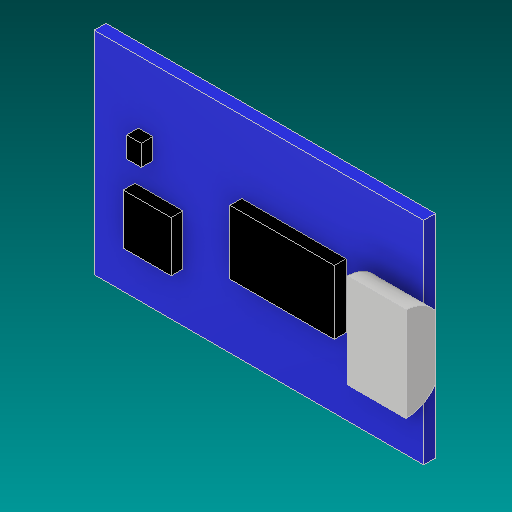
# Autodesk Inventor part: Regulador
Saved by Autodesk Inventor 2019 (Build 230136000, 136)
## iProperties
Created: 2020-01-17
Part Number: Regulador
Material: Generic
Document SubType Name: Modeling
Designer: Santiago
Density: 1 g/cm^3
Appearance: Default
Author: Santiago
Autodesk Inventor part; units mm, degrees
ref_plane "YZ Plane" through (0, 0, 0) normal (1, 0, 0) x (0, 1, 0)
ref_plane "XZ Plane" through (0, 0, 0) normal (0, 1, 0) x (-1, 0, 0)
ref_plane "XY Plane" through (0, 0, 0) normal (0, 0, 1) x (1, 0, 0)
sketch "Sketch1" plane through (0, 0, 0) normal (0, 0, 1) x (1, 0, 0)
  line L0 (0, 0) -> (28, 0)
  line L1 (28, 0) -> (28, 18)
  line L2 (28, 18) -> (0, 18)
  line L3 (0, 18) -> (0, 0)
  dimension "d0" = 28
  dimension "d1" = 18
  dimension "d2" = 28
  constraints: 8 end point, 2 perpendicular, 1 horizontal
  measures "d0" distance of L0.start L0.end
  measures "d1" distance of L0.end L1.end
  measures "d2" distance of L1.end L2.end
extrude "Extrusion1" add sketch "Sketch1" along normal blind 1
sketch "Sketch2" plane through (0, 0, 1) normal (0, 0, 1) x (1, 0, 0)
  line L0 (21.3992, 11.8771) -> (21.3992, 6.4359)
  line L1 (21.3992, 6.4359) -> (12.5353, 6.4359)
  line L2 (12.5353, 6.4359) -> (12.5353, 11.8771)
  line L3 (12.5353, 11.8771) -> (21.3992, 11.8771)
  line L4 (3.7591, 12.6669) -> (3.7591, 10.8901)
  line L5 (3.7591, 10.8901) -> (4.997, 10.8901)
  line L6 (4.997, 10.8901) -> (4.997, 12.6669)
  line L7 (4.997, 12.6669) -> (3.7591, 12.6669)
  line L8 (3.4697, 8.4681) -> (7.5353, 8.4681)
  line L9 (7.5353, 8.4681) -> (7.5353, 4.1843)
  line L10 (7.5353, 4.1843) -> (3.4697, 4.1843)
  line L11 (3.4697, 4.1843) -> (3.4697, 8.4681)
  point P0 (0, 0)
  constraints: 24 end point, 9 perpendicular, 2 vertical, 1 horizontal
extrude "Extrusion2" add sketch "Sketch2" along normal blind 1
sketch "Sketch3" plane through (28, 0, 0) normal (1, 0, 0) x (0, 0, -1)
  line L0 (-1, 6.4359) -> (-1, 11.8771) projected
  line L1 (-1, 9.1565) -> (-3.5, 9.1565)
  line L2 (-3.5, 9.1565) -> (-3.5, 13.1565)
  line L3 (-3.5, 13.1565) -> (-3.5, 5.1565)
  line L4 (-2, 8.4681) -> (-2, 4.1843) projected
  line L5 (-2, 11.8771) -> (-2, 6.4359) projected
  line L6 (-2, 9.1565) -> (-2, 6.3262)
  arc A0 (-3.5, 5.1565) -> (-1, 6.4359) centre (-3.4729, 8.1858) ccw
  arc A1 (-1, 11.8771) -> (-3.5, 13.1565) centre (-3.6026, 9.8737) ccw
  line L7 (-1, 6.4359) -> (-1, 11.8771)
  point P0 (0, 0)
  dimension "d7" = 2.5
  dimension "d8" = 4
  dimension "d9" = 8
  constraints: 10 end point, 4 point on circle, 3 midpoint, 2 centre point, 2 collinear, 1 horizontal, 1 point on line, 1 vertical
  measures "d7" distance of L1.start L1.end
  measures "d8" distance of L1.end L2.end
  measures "d9" distance of L2.end L3.end
extrude "Extrusion3" add sketch "Sketch3" along normal blind 1
sketch "Sketch4" plane through (28, 0, 0) normal (-1, 0, 0) x (0, 0, 1)
  arc A0 (3.5, 13.1565) -> (1, 11.8771) centre (3.6026, 9.8737) ccw projected
  line L0 (1, 6.4359) -> (1, 11.8771) projected
  arc A1 (1, 6.4359) -> (3.5, 5.1565) centre (3.4729, 8.1858) ccw projected
  line L1 (3.5, 13.1565) -> (3.5, 5.1565) projected
  point P0 (0, 0)
extrude "Extrusion4" add sketch "Sketch4" along normal blind 4
body "Solid1"
